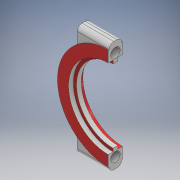
# Autodesk Inventor part: reverse gear lower trap
Saved by Autodesk Inventor 2017 (Build 210142000, 142)
## iProperties
Created: 2018-11-16
Part Number: reverse gear lower trap
Material: Generic
Document SubType Name: Modeling
Designer: User
Density: 1 g/cm^3
Appearance: Default
Author: User
Autodesk Inventor part; units mm, degrees
ref_plane "YZ Plane" through (0, 0, 0) normal (1, 0, 0) x (0, 1, 0)
ref_plane "XZ Plane" through (0, 0, 0) normal (0, 1, 0) x (-1, 0, 0)
ref_plane "XY Plane" through (0, 0, 0) normal (0, 0, 1) x (1, 0, 0)
sketch "Sketch1" plane through (0, 0, 0) normal (0, 1, 0) x (-1, 0, 0)
  arc A0 (0, -16) -> (0, 16) centre (0, 0) ccw
  arc A1 (0, -11.5) -> (0, 11.5) centre (0, 0) ccw
  line L0 (0, 16) -> (0, 11.5)
  line L1 (0, -11.5) -> (0, -16)
  arc A2 (0, -12.5) -> (0, 12.5) centre (0, 0) ccw
  dimension "d0" = 32
  dimension "d1" = 23
  dimension "d2" = 0
  dimension "d3" = 0
  dimension "d4" = 25
  dimension "d5" = 0
  dimension "d6" = 16
  dimension "d7" = 0
  dimension "d8" = 16
  constraints: 6 point on circle, 4 end point, 3 centre point, 2 point on line, 2 vertical, 1 coincident, 1 concentric
  measures "d0" diameter of A0
  measures "d1" diameter of A1
  measures "d2" distance between parallel lines of L0 L1
  measures "d3" distance from line of A0.centre L0
  measures "d4" diameter of A2
  measures "d5" distance from line of point (0, 0) L0
  measures "d6" distance of point (0, 0) L0.start
  measures "d7" distance from line of point (0, 0) L0
  measures "d8" distance of point (0, 0) L0.start
extrude "Extrusion1" add sketch "Sketch1" along normal mid plane 4.5 contours L1 A2 L0 A0
extrude "Extrusion2" add sketch "Sketch1" along normal mid plane 1.5 contours L1 A1 L0 A2
sketch "Sketch3" plane through (0, -2.25, -16) normal (1, 0, 0) x (0, 0, -1)
  line L0 (-32, 4.5) -> (-28.5, 4.5)
  line L1 (-30.25, 4.5) -> (-30.25, 4.25)
  line L2 (-28.5, 0) -> (-32, 0)
  line L3 (-30.25, 0) -> (-30.25, 0.25)
  line L4 (-28.5, 3) -> (-28.5, 4.5)
  line L5 (-28.5, 4.25) -> (-32, 4.25)
  line L6 (-33.5, 2.75) -> (-33.5, 1.75)
  line L7 (-32, 0.25) -> (-28.5, 0.25)
  line L8 (-28.5, 0.25) -> (-28.5, 4.25)
  arc A0 (-32, 4.25) -> (-33.5, 2.75) centre (-32, 2.75) ccw
  arc A1 (-33.5, 1.75) -> (-32, 0.25) centre (-32, 1.75) ccw
  circle A2 centre (-30.2, 2.25) radius 1.5
  line L9 (-32, 4.5) -> (-32, 0)
  line L10 (-3.5, 1.5) -> (-28.5, 1.5)
  line L11 (-3.5, 4.25) -> (0, 4.25)
  circle A3 centre (-1.8, 2.25) radius 1.5
  arc A4 (1.5, 2.75) -> (0, 4.25) centre (0, 2.75) ccw
  arc A5 (0, 0.25) -> (1.5, 1.75) centre (0, 1.75) ccw
  line L12 (1.5, 2.75) -> (1.5, 1.75)
  line L13 (-3.5, 3) -> (-3.5, 4.25)
  line L14 (0, 0.25) -> (-3.5, 0.25)
  line L15 (-3.5, 0.25) -> (-3.5, 4.25)
  line L16 (-4.5, 3) -> (-4.5, 1.5)
  line L17 (-27.5, 3) -> (-4.5, 3)
  line L18 (-27.5, 1.5) -> (-27.5, 3)
  line L19 (-4.5, 1.5) -> (-27.5, 1.5)
  point P0 (-16, 2.25)
  dimension "d13" = 3
  dimension "d14" = 5
  dimension "d15" = 2.7
  dimension "d16" = 2.7
  dimension "d17" = 90
  dimension "d18" = 90
  dimension "d19" = 90
  dimension "d20" = 6
  dimension "d21" = 2.75
  dimension "d22" = 1.25
  dimension "d23" = 1
  dimension "d24" = 0
  dimension "d25" = 24
  dimension "d26" = 27.5
  dimension "d27" = 29
  dimension "d28" = 1.5
  dimension "d29" = 3
  dimension "d30" = 25.75
  dimension "d31" = 0.75
  dimension "d32" = 1.5
  dimension "d33" = 1.5
  dimension "d34" = 24
  dimension "d35" = 0.75
  dimension "d36" = 2.75
  dimension "d37" = 1.25
  constraints: 40 end point, 10 tangent, 9 parallel, 8 point on circle, 6 centre point, 5 equal radius, 2 horizontal, 2 midpoint, 1 perpendicular, 1 point on line, 1 vertical
  measures "d13" diameter of A2
  measures "d14" distance from line of L10.start L12
  measures "d15" distance from line of L18 A2.centre
  measures "d16" distance from line of L16 A3.centre
  measures "d17" angle of L19 L13
  measures "d18" angle of L19 L4
  measures "d19" angle of L19 L1
  measures "d20" distance between parallel lines of L16 L12
  measures "d21" distance between parallel lines of L19 L11
  measures "d22" distance between parallel lines of L19 L14
  measures "d23" distance between parallel lines of L16 L15
  measures "d24" distance between parallel lines of L19 L10
  measures "d25" distance between parallel lines of L16 L8
  measures "d26" distance between parallel lines of L16 L9
  measures "d27" distance between parallel lines of L16 L6
  measures "d28" distance between parallel lines of L19 L2
  measures "d29" distance between parallel lines of L19 L0
  measures "d30" distance between parallel lines of L3 L16
  measures "d31" distance from line of A3.centre L19
  measures "d32" distance from line of L13.start L19
  measures "d33" distance from line of L4.start L19
  measures "d34" distance from line of L10.end L16
  measures "d35" distance from line of A2.centre L19
  measures "d36" distance from line of L1.end L19
  measures "d37" distance from line of L3.end L19
extrude "Extrusion3" add sketch "Sketch3" against normal blind 10 contours L15 L13 L11 A4 L12 A5 L14 | L9 A1 L6 A0 | L5 L4 L8 L7 L9
extrude "Extrusion4" cut sketch "Sketch3" against normal blind 10 contours A2 | A3
body "Solid1"
